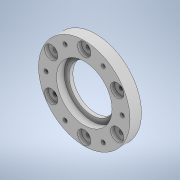
# Autodesk Inventor part: 28521_Bearing_Holder
Saved by Autodesk Inventor 2020 (Build 240168000, 168)
## iProperties
Created: 2020-01-24
Part Number: 28521_Bearing_Holder
Material: Generic
Document SubType Name: Modeling
Designer: srini
Density: 1 g/cm^3
Appearance: Default
Author: srini
Autodesk Inventor part; units mm, degrees
ref_plane "YZ Plane" through (0, 0, 0) normal (1, 0, 0) x (0, 1, 0)
ref_plane "XZ Plane" through (0, 0, 0) normal (0, 1, 0) x (-1, 0, 0)
ref_plane "XY Plane" through (0, 0, 0) normal (0, 0, 1) x (1, 0, 0)
sketch "Sketch1" plane through (0, 0, 0) normal (0, 0, 1) x (1, 0, 0)
  circle A0 centre (0, 0) radius 76.2
  circle A1 centre (0, 63.5) radius 3.3734
  circle A2 centre (0, 0) radius 38.1
  circle A3 centre (-31.75, 54.9926) radius 3.3734
  circle A4 centre (-54.9926, 31.75) radius 3.3734
  circle A5 centre (-63.5, 0) radius 3.3734
  circle A6 centre (-54.9926, -31.75) radius 3.3734
  circle A7 centre (-31.75, -54.9926) radius 3.3734
  circle A8 centre (0, -63.5) radius 3.3734
  circle A9 centre (31.75, -54.9926) radius 3.3734
  circle A10 centre (54.9926, -31.75) radius 3.3734
  circle A11 centre (63.5, 0) radius 3.3734
  circle A12 centre (54.9926, 31.75) radius 3.3734
  circle A13 centre (31.75, 54.9926) radius 3.3734
  dimension "d0" = 63.5
  dimension "d1" = 152.4
  dimension "d2" = 6.7469
  dimension "d3" = 76.2
  dimension "d6" = 360
  constraints: 14 centre point, 2 coincident, 1 vertical alignment, 25 other
  measures "d0" distance of point (0, 0) A1.centre
  measures "d1" diameter of A0
  measures "d2" diameter of A1
  measures "d3" diameter of A2
extrude "Extrusion1" add sketch "Sketch1" along normal blind 6.35
sketch "Sketch2" plane through (0, 0, 6.35) normal (0, 0, 1) x (1, 0, 0)
  circle A0 centre (0, 0) radius 46.2375
  circle A1 centre (0, 0) radius 52.5875
  dimension "d10" = 92.475
  dimension "d11" = 6.35
  constraints: 2 centre point, 2 coincident
  measures "d10" diameter of A0
  measures "d11" radial gap between concentric circles of A0 A1
extrude "Extrusion2" add sketch "Sketch2" along normal blind 12.7
sketch "Sketch3" plane through (0, 0, 6.35) normal (0, 0, 1) x (1, 0, 0)
  circle A0 centre (0, 63.5) radius 3.3734 projected
  circle A1 centre (-54.9926, 31.75) radius 3.3734 projected
  circle A2 centre (54.9926, -31.75) radius 3.3734 projected
  circle A3 centre (0, -63.5) radius 3.3734 projected
  circle A4 centre (-63.5, 0) radius 3.3734 projected
  circle A5 centre (31.75, 54.9926) radius 3.3734 projected
  circle A6 centre (-31.75, 54.9926) radius 3.3734 projected
  circle A7 centre (54.9926, 31.75) radius 3.3734 projected
  circle A8 centre (-31.75, -54.9926) radius 3.3734 projected
  circle A9 centre (-54.9926, -31.75) radius 3.3734 projected
  circle A10 centre (31.75, -54.9926) radius 3.3734 projected
  circle A11 centre (63.5, 0) radius 3.3734 projected
  circle A12 centre (0, 0) radius 76.2 projected
  circle A13 centre (0, 0) radius 52.5875 projected
extrude "Extrusion3" add sketch "Sketch3" along normal blind 12.7
sketch "Sketch4" plane through (0, 0, 19.05) normal (0, 0, 1) x (1, 0, 0)
  circle A0 centre (0, 63.5) radius 3.3734 construction
  circle A1 centre (0, 63.5) radius 11.1125
  circle A2 centre (-54.9926, 31.75) radius 11.1125
  circle A3 centre (-54.9926, -31.75) radius 11.1125
  circle A4 centre (0, -63.5) radius 11.1125
  circle A5 centre (54.9926, -31.75) radius 11.1125
  circle A6 centre (54.9926, 31.75) radius 11.1125
  point P0 (0, 0)
  dimension "d16" = 22.225
  dimension "d19" = 360
  constraints: 6 centre point, 6 coincident, 19 other
  measures "d16" diameter of A1
extrude "Extrusion4" cut sketch "Sketch4" against normal blind 6.35
body "Solid1"
